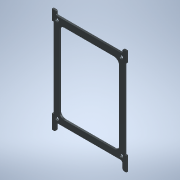
# Autodesk Inventor part: back bracer
Saved by Autodesk Inventor 2022 (Build 260153000, 153)
## iProperties
Created: 2021-05-28
Part Number: back bracer
Material: Iron, Cast
Document SubType Name: Modeling
Designer: benka
Density: 7.15 g/cm^3
Appearance: Iron Gray
Author: benka
Autodesk Inventor part; units mm, degrees
ref_plane "YZ Plane" through (0, 0, 0) normal (1, 0, 0) x (0, 1, 0)
ref_plane "XZ Plane" through (0, 0, 0) normal (0, 1, 0) x (-1, 0, 0)
ref_plane "XY Plane" through (0, 0, 0) normal (0, 0, 1) x (1, 0, 0)
sketch "Sketch1" plane through (0, 0, 0) normal (0, 0, 1) x (1, 0, 0)
  line L0 (98.9439, 111.9936) -> (98.9439, -112.0064)
  line L1 (103.9439, 111.9936) -> (98.9439, 111.9936)
  line L2 (103.9439, 141.2436) -> (103.9439, 111.9936)
  line L3 (83.9439, -97.0105) -> (83.9439, 96.9895)
  line L4 (-99.0561, 111.9936) -> (-104.0561, 111.9936)
  line L5 (-104.0561, 111.9936) -> (-104.0561, 141.2436)
  line L6 (-99.0561, -112.0064) -> (-99.0561, 111.9936)
  line L7 (-84.0561, 96.9895) -> (-84.0561, -97.0105)
  line L8 (-69.0561, 111.9895) -> (68.9439, 111.9895)
  line L9 (68.9439, -112.0105) -> (-69.0561, -112.0105)
  line L10 (103.9439, -112.0064) -> (98.9439, -112.0064)
  line L11 (103.9439, -152.0064) -> (103.9439, -112.0064)
  line L12 (-99.0561, -112.0064) -> (-104.0561, -112.0064)
  line L13 (-104.0561, -112.0064) -> (-104.0561, -152.0064)
  arc A0 (-98.0561, -152.0064) -> (-93.0561, -147.0064) centre (-98.0561, -147.0064) ccw
  line L14 (103.9439, -152.0064) -> (97.9439, -152.0064)
  line L15 (-88.0561, -129.0585) -> (74.9433, -129.0585)
  line L16 (-104.0561, -152.0064) -> (-98.0561, -152.0064)
  line L17 (74.9433, -129.0585) -> (87.9439, -129.0585)
  line L18 (92.9439, -134.0585) -> (92.9439, -147.0064)
  arc A1 (92.9439, -147.0064) -> (97.9439, -152.0064) centre (97.9439, -147.0064) ccw
  arc A2 (92.9439, -134.0585) -> (87.9439, -129.0585) centre (87.9439, -134.0585) ccw
  line L19 (-104.0561, 141.2436) -> (-96.0561, 141.2436)
  line L20 (-93.0561, 138.2436) -> (-93.0561, 133.2436)
  arc A3 (-93.0561, 138.2436) -> (-96.0561, 141.2436) centre (-96.0561, 138.2436) ccw
  line L21 (-93.0561, -147.0064) -> (-93.0561, -134.0585)
  arc A4 (-88.0561, -129.0585) -> (-93.0561, -134.0585) centre (-88.0561, -134.0585) ccw
  line L22 (103.9439, 141.2436) -> (95.9439, 141.2436)
  arc A5 (95.9439, 141.2436) -> (92.9439, 138.2436) centre (95.9439, 138.2436) ccw
  arc A6 (-69.0561, 111.9895) -> (-84.0561, 96.9895) centre (-69.0561, 96.9895) ccw
  arc A7 (-84.0561, -97.0105) -> (-69.0561, -112.0105) centre (-69.0561, -97.0105) ccw
  arc A8 (68.9439, -112.0105) -> (83.9439, -97.0105) centre (68.9439, -97.0105) ccw
  arc A9 (83.9439, 96.9895) -> (68.9439, 111.9895) centre (68.9439, 96.9895) ccw
  line L23 (92.9439, 138.2436) -> (92.9439, 133.2436)
  line L24 (89.9439, 130.2436) -> (-90.0561, 130.2436)
  arc A10 (89.9439, 130.2436) -> (92.9439, 133.2436) centre (89.9439, 133.2436) ccw
  arc A11 (-93.0561, 133.2436) -> (-90.0561, 130.2436) centre (-90.0561, 133.2436) ccw
  circle A12 centre (89.9439, 119.8071) radius 5
  circle A13 centre (-90.0561, 119.8071) radius 5
  circle A14 centre (89.9439, -118.7922) radius 5
  circle A15 centre (-90.0561, -118.7922) radius 5
  point P0 (83.9439, 91.9897)
  point P1 (83.9439, -92.0105)
  point P2 (53.9441, 111.9895)
  point P3 (53.9441, -112.0105)
  point P4 (-84.0561, 91.9895)
  point P5 (-64.0561, -112.0105)
  point P6 (-84.0561, -92.0105)
  point P7 (-64.0561, 111.9895)
  point P8 (93.9439, -152.0064)
  point P9 (-99.0561, -111.9897)
  point P10 (98.9427, -111.9902)
  point P11 (-91.5561, -141.2436)
  point P12 (-91.5561, -141.2564)
  point P13 (-91.5556, -141.2564)
  point P14 (-93.0561, -130.0064)
  point P15 (-93.0561, 141.2436)
  point P16 (-91.5561, 136.2791)
  point P17 (92.9439, 141.2436)
  dimension "d29" = 198
  dimension "d30" = 5
  dimension "d31" = 5
  dimension "d32" = 5
  dimension "d33" = 5
  dimension "d34" = 15
  dimension "d35" = 15
  dimension "d36" = 224
  dimension "d37" = 224
  dimension "d38" = 40
  dimension "d39" = 40
  dimension "d42" = 208
  dimension "d43" = 208
  dimension "d45" = 6
  dimension "d48" = 5
  dimension "d57" = 3
  dimension "d60" = 5
  dimension "d62" = 3
  dimension "d64" = 15
  dimension "d65" = 15
  dimension "d66" = 5
  dimension "d67" = 5
  dimension "d69" = 3
  dimension "d70" = 8
  dimension "d71" = 8
  dimension "d72" = 6
  dimension "d73" = 10
  dimension "d74" = 10
  dimension "d75" = 10
  dimension "d76" = 10
  constraints: 50 end point, 24 point on circle, 21 tangent, 16 centre point, 13 point on line, 8 perpendicular, 7 horizontal, 4 equal radius, 3 parallel, 2 collinear, 2 vertical, 1 other
  measures "d29" distance between parallel lines of L0 L6
  measures "d30" distance between parallel lines of L6 L5
  measures "d31" distance between parallel lines of L2 L0
  measures "d32" distance between parallel lines of L6 L13
  measures "d33" distance between parallel lines of L11 L0
  measures "d34" distance between parallel lines of L0 L3
  measures "d35" distance between parallel lines of L7 L6
  measures "d36" distance between parallel lines of L12 L4
  measures "d37" distance between parallel lines of L1 L10
  measures "d38" distance between parallel lines of L12 L16
  measures "d39" distance between parallel lines of L10 L14
  measures "d42" distance between parallel lines of L2 L5
  measures "d43" distance between parallel lines of L11 L13
  measures "d45" distance of L13.end L16.end
  measures "d48" radius of A1
  measures "d57" radius of A3
  measures "d60" radius of A4
  measures "d62" radius of A5
  measures "d64" radius of A6
  measures "d65" radius of A7
  measures "d66" distance of L23.end L23.start
  measures "d67" distance of L20.end L20.start
  measures "d69" radius of A10
  measures "d70" distance of L2.start L22.end
  measures "d71" distance of L5.end L19.end
  measures "d72" distance of L14.start L14.end
  measures "d73" diameter of A12
  measures "d74" diameter of A13
  measures "d75" diameter of A14
  measures "d76" diameter of A15
extrude "Extrusion1" add sketch "Sketch1" along normal blind 5
body "Solid1"
